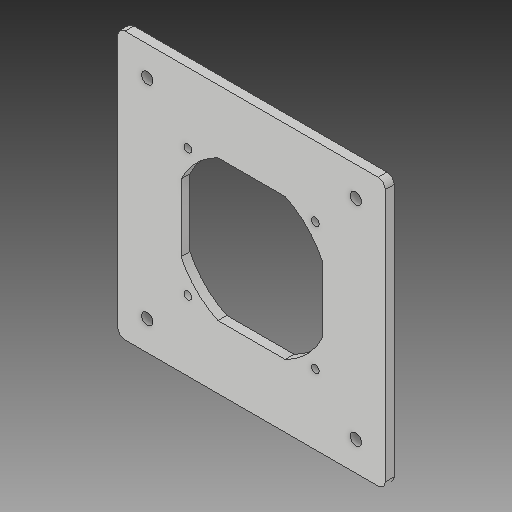
# Autodesk Inventor part: TablaSoporte1
Saved by Autodesk Inventor 2017 (Build 210142000, 142)
## iProperties
Part Number: TablaSoporte1
Material: Genérico
Document SubType Name: Modeling
Designer: Leonardo
Density: 1 g/cm^3
Appearance: Valor por defecto
Mass: 83.4941 g
Surface Area: 383.902 cm^2
Volume: 83.4941 cm^3
Author: Leonardo
Autodesk Inventor part; units mm, degrees
ref_plane "YZ Plane" through (0, 0, 0) normal (1, 0, 0) x (0, 1, 0)
ref_plane "XZ Plane" through (0, 0, 0) normal (0, 1, 0) x (-1, 0, 0)
ref_plane "XY Plane" through (0, 0, 0) normal (0, 0, 1) x (1, 0, 0)
sketch "Boceto1" plane through (0, 0, 0) normal (0, 0, 1) x (1, 0, 0)
  line L0 (71, 32.2855) -> (-71, 32.2855)
  line L1 (-75, 28.2855) -> (-75, -113.7145)
  line L2 (-71, -117.7145) -> (71, -117.7145)
  line L3 (75, -113.7145) -> (75, 28.2855)
  line L4 (75, 32.2855) -> (-75, -117.7145) construction
  line L5 (-75, 32.2855) -> (75, -117.7145) construction
  circle A0 centre (35.75, -6.9645) radius 2.2 projected
  circle A1 centre (35.75, -78.4645) radius 2.2 projected
  circle A2 centre (-35.75, -78.4645) radius 2.2 projected
  circle A3 centre (-35.75, -6.9645) radius 2.2 projected
  arc A4 (39.55, -23.817) -> (18.8975, -3.1645) centre (0, -42.7145) ccw projected
  arc A5 (18.8975, -82.2645) -> (39.55, -61.612) centre (0, -42.7145) ccw projected
  arc A6 (-39.55, -61.612) -> (-18.8975, -82.2645) centre (0, -42.7145) ccw projected
  arc A7 (-18.8975, -3.1645) -> (-39.55, -23.817) centre (0, -42.7145) ccw projected
  line L6 (18.8975, -3.1645) -> (-18.8975, -3.1645)
  line L7 (39.55, -23.817) -> (39.55, -61.612)
  line L8 (18.8975, -82.2645) -> (-18.8975, -82.2645)
  line L9 (-39.55, -61.612) -> (-39.55, -23.817)
  line L10 (71, -117.7145) -> (42, -117.7145)
  line L11 (75, -84.7145) -> (75, -113.7145)
  line L12 (71, 32.2855) -> (42, 32.2855)
  line L13 (75, -0.7145) -> (75, 28.2855)
  line L14 (-71, 32.2855) -> (-42, 32.2855)
  line L15 (-75, -0.7145) -> (-75, 28.2855)
  line L16 (-71, -117.7145) -> (-42, -117.7145)
  line L17 (-75, -84.7145) -> (-75, -113.7145)
  line L18 (42, 32.2855) -> (75, -0.7145) construction
  line L19 (75, -84.7145) -> (42, -117.7145) construction
  line L20 (-75, -84.7145) -> (-42, -117.7145) construction
  line L21 (-42, 32.2855) -> (-75, -0.7145) construction
  circle A8 centre (-58.5, 15.7855) radius 3.175
  circle A9 centre (-58.5, -101.2145) radius 3.175
  circle A10 centre (58.5, 15.7855) radius 3.175
  circle A11 centre (58.5, -101.2145) radius 3.175
  arc A12 (75, 28.2855) -> (71, 32.2855) centre (71, 28.2855) ccw
  arc A13 (71, -117.7145) -> (75, -113.7145) centre (71, -113.7145) ccw
  arc A14 (-75, -113.7145) -> (-71, -117.7145) centre (-71, -113.7145) ccw
  arc A15 (-71, 32.2855) -> (-75, 28.2855) centre (-71, 28.2855) ccw
  arc A16 (18.8975, -82.2645) -> (39.55, -61.612) centre (0, -42.7145) ccw
  arc A17 (-39.55, -61.612) -> (-18.8975, -82.2645) centre (0, -42.7145) ccw
  arc A18 (39.55, -23.817) -> (18.8975, -3.1645) centre (0, -42.7145) ccw
  arc A19 (-18.8975, -3.1645) -> (-39.55, -23.817) centre (0, -42.7145) ccw
  point P0 (0, 0)
  dimension "d10" = 6.35
  dimension "d11" = 6.35
  dimension "d12" = 6.35
  dimension "d13" = 6.35
  dimension "d14" = 4
  constraints: 44 end point, 18 point on circle, 12 centre point, 8 point on line, 8 tangent, 6 horizontal, 6 perpendicular, 4 midpoint, 3 equal radius, 2 parallel, 1 coincident
  measures "d10" diameter of A8
  measures "d11" diameter of A9
  measures "d12" diameter of A10
  measures "d13" diameter of A11
  measures "d14" radius of A12
extrude "Extrusión1" add sketch "Boceto1" along normal blind 5
